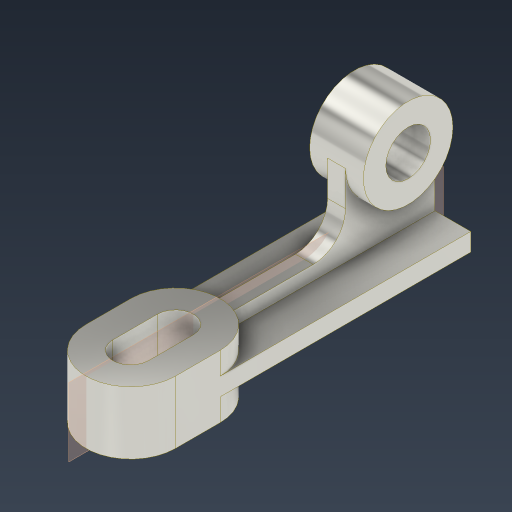
# Autodesk Inventor part: Peça teste2
Saved by Autodesk Inventor 2024 (Build 280153000, 153)
## iProperties
Created: 2024-02-12
Part Number: Peça teste2
Material: Prata
Document SubType Name: Modeling
Designer: Administrator
Density: 10.49 g/cm^3
Appearance: Prata
Author: Administrator
Autodesk Inventor part; units mm, degrees
ref_plane "YZ Plane" through (0, 0, 0) normal (1, 0, 0) x (0, 1, 0)
ref_plane "XZ Plane" through (0, 0, 0) normal (0, 1, 0) x (-1, 0, 0)
ref_plane "XY Plane" through (0, 0, 0) normal (0, 0, 1) x (1, 0, 0)
sketch "Esboço1" plane through (0, 0, 0) normal (0, 1, 0) x (-1, 0, 0)
  line L0 (-25, 76.25) -> (25, 76.25)
  line L1 (25, 76.25) -> (25, -76.25)
  line L2 (25, -76.25) -> (-25, -76.25)
  line L3 (-25, -76.25) -> (-25, 76.25)
  line L4 (-25, 76.25) -> (25, -76.25) construction
  line L5 (25, 76.25) -> (-25, -76.25) construction
  line L6 (0, 88.75) -> (0, 63.75) construction
  line L7 (-25, 88.75) -> (-25, 63.75)
  line L8 (25, 63.75) -> (25, 88.75)
  arc A0 (25, 88.75) -> (-25, 88.75) centre (0, 88.75) ccw
  arc A1 (-25, 63.75) -> (25, 63.75) centre (0, 63.75) ccw
  point P0 (0, 0)
  point P1 (0, 76.25)
  point P2 (0, -76.25)
  point P3 (0, 113.75)
  dimension "d0" = 190
  dimension "d1" = 50
  dimension "d2" = 25
  constraints: 20 end point, 5 midpoint, 5 point on circle, 4 tangent, 3 parallel, 2 centre point, 1 collinear, 1 horizontal, 1 perpendicular, 1 vertical
  measures "d0" distance of point (0, -76.25) point (0, 113.75)
  measures "d1" distance between parallel lines of L7 L8
  measures "d2" distance of L6.end L6.start
extrude "Extrusão1" add sketch "Esboço1" along normal mid plane 35 contours L7 A0 L8 L0 | L0 L1 A1 L3
extrude "Extrusão2" add sketch "Esboço1" along normal mid plane 10 contours A1 L1 L2 L3
ref_plane "Plano de trabalho1" through (0, -17.5, 88.75) normal (1, 0, 0) x (0, 0, -1)
sketch "Esboço2" plane through (0, -17.5, 88.75) normal (1, 0, 0) x (0, 0, -1)
  circle A0 centre (140, 68) radius 25
  line L0 (165, 12.5) -> (165, 22.5) projected
  line L1 (165, 12.5) -> (25, 12.5) projected
  point P0 (88.75, 17.5)
  dimension "d7" = 50
  dimension "d10" = 55.5
  constraints: 1 centre point, 1 tangent
  measures "d7" diameter of A0
  measures "d10" distance from line of L1 A0.centre
extrude "Extrusão3" add sketch "Esboço2" along normal mid plane 30
sketch "Esboço5" plane through (0, -17.5, 88.75) normal (1, 0, 0) x (0, 0, -1)
  line L0 (25, 22.5) -> (165, 22.5) projected
  line L1 (165, 22.5) -> (165, 68)
  circle A0 centre (140, 68) radius 25 projected
  line L2 (165, 22.5) -> (14.8808, 22.5)
  line L3 (14.8808, 22.5) -> (14.8808, 30.5)
  line L4 (14.8808, 30.5) -> (97, 30.5)
  line L5 (115, 48.5) -> (115, 68)
  arc A1 (97, 30.5) -> (115, 48.5) centre (97, 48.5) ccw
  point P0 (88.75, 17.5)
  dimension "d11" = 8
  dimension "d12" = 18
  constraints: 10 end point, 4 point on circle, 4 tangent, 2 perpendicular, 1 centre point, 1 horizontal
  measures "d11" distance between parallel lines of L0 L4
  measures "d12" radius of A1
extrude "Extrusão4" add sketch "Esboço5" along normal mid plane 10 contours L2 L3 L4 A1 L5 A0 L1 L0
sketch "Esboço6" plane through (15, 50.5, -51.25) normal (1, 0, 0) x (0, 0, -1)
  circle A0 centre (0, 0) radius 25 projected
  point P0 (-51.25, -50.5)
  constraints: 1 coincident
hole "Furo1" at (15, 50.5, -51.25) direction (-1, 0, 0) diameter 25 end through all
sketch "Esboço7" plane through (0, 17.5, 0) normal (0, 1, 0) x (1, 0, 0)
  line L0 (25, -88.75) -> (25, -63.75) projected
  arc A0 (25, -63.75) -> (-25, -63.75) centre (0, -63.75) ccw projected
  line L1 (-25, -63.75) -> (-25, -88.75) projected
  arc A1 (-25, -88.75) -> (25, -88.75) centre (0, -88.75) ccw projected
  line L2 (10, -88.75) -> (10, -63.75)
  arc A2 (10, -63.75) -> (-10, -63.75) centre (0, -63.75) ccw
  line L3 (-10, -63.75) -> (-10, -88.75)
  arc A3 (-10, -88.75) -> (10, -88.75) centre (0, -88.75) ccw
  point P0 (0, 0)
  dimension "d22" = 20
  constraints: 4 end point, 4 point on circle, 2 centre point, 3 other
  measures "d22" distance between parallel lines of L2 L3
extrude "Extrusão5" cut sketch "Esboço7" against normal through all contours A3 L3 A2 L2
